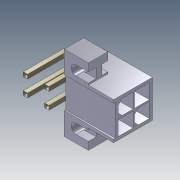
# Autodesk Inventor part: minifit-2x2rb
Saved by Autodesk Inventor 2015 SP1 (Build 190203100, 203)
## iProperties
Created: 2016-02-27
Part Number: minifit-2x2rb
Material: Generic
Document SubType Name: Modeling
Designer: Kostic
Density: 1 g/cm^3
Appearance: Default
Author: Kostic
Autodesk Inventor part; units mm, degrees
ref_plane "YZ Plane" through (0, 0, 0) normal (1, 0, 0) x (0, 1, 0)
ref_plane "XZ Plane" through (0, 0, 0) normal (0, 1, 0) x (-1, 0, 0)
ref_plane "XY Plane" through (0, 0, 0) normal (0, 0, 1) x (1, 0, 0)
sketch "Sketch1" plane through (0, 0, 0) normal (1, 0, 0) x (0, 1, 0)
  line L0 (0, 0) -> (10, 0)
  line L1 (10, 0) -> (10, -9.6)
  line L2 (10, -9.6) -> (0, -9.6)
  line L3 (0, -9.6) -> (0, 0)
  dimension "d0" = 10
  dimension "d1" = 9.6
  constraints: 8 end point, 2 parallel, 1 horizontal, 1 perpendicular
  measures "d0" distance of L1.end L2.end
  measures "d1" distance of L0.end L1.end
extrude "Extrusion1" add sketch "Sketch1" along normal blind 12.7
sketch "Sketch2" plane through (0, 0, -9.6) normal (0, -1, 0) x (1, 0, 0)
  line L0 (0, 14.55) -> (6.2, 14.55)
  line L1 (6.2, 14.55) -> (6.2, -4.95)
  line L2 (6.2, -4.95) -> (0, -4.95)
  line L3 (0, -4.95) -> (0, 14.55)
  line L4 (0, 0) -> (12.7, 0) projected
  point P0 (0, 9.6)
  dimension "d4" = 6.2
  dimension "d5" = 19.5
  dimension "d6" = 4.95
  constraints: 8 end point, 2 parallel, 1 horizontal, 1 perpendicular
  measures "d4" distance of L1.end L2.end
  measures "d5" distance of L0.end L1.end
  measures "d6" distance between parallel lines of L4 L2
extrude "Extrusion2" add sketch "Sketch2" against normal blind 5
hole "Hole1" at (3, 5, -11.3) direction (0, -1, 0) diameter 2.5 end through all
hole "Hole2" at (3, 5, 1.7) direction (0, -1, 0) diameter 2.5 end through all
sketch "Sketch3" plane through (0, 5, -9.6) normal (0, 1, 0) x (1, 0, 0)
  circle A0 centre (3, 1.7) radius 1.25 projected
  line L0 (3, 0.45) -> (6.2, 0.45)
  line L1 (6.2, 0.45) -> (6.2, 2.95)
  line L2 (6.2, 2.95) -> (3, 2.95)
  line L3 (3, 2.95) -> (3, 0.45)
  circle A1 centre (3, -11.3) radius 1.25 projected
  line L4 (3, -12.55) -> (6.2, -12.55)
  line L5 (6.2, -12.55) -> (6.2, -10.05)
  line L6 (6.2, -10.05) -> (3, -10.05)
  line L7 (3, -10.05) -> (3, -12.55)
  point P0 (0, -9.6)
  dimension "d27" = 3.2
  dimension "d28" = 2.5
  dimension "d29" = 3.2
  dimension "d30" = 2.5
  constraints: 16 end point, 4 parallel, 2 horizontal, 2 perpendicular, 2 vertical alignment, 1 point on line, 2 other
  measures "d27" distance of L2.end L1.end
  measures "d28" distance of L1.end L0.end
  measures "d29" distance of L6.end L5.end
  measures "d30" distance of L5.end L4.end
extrude "Extrusion3" cut sketch "Sketch3" against normal blind 1.5 contours A0 L3 | A0 L2 L1 L0 | A1 L7 | A1 L6 L5 L4 picked at (3.2598, 2.0258) picked at (3.5112, -11.0402)
sketch "Sketch4" plane through (12.7, 0, 0) normal (1, 0, 0) x (0, 0, -1)
  line L0 (0.8, 9.2) -> (4.6, 9.2)
  line L1 (4.6, 9.2) -> (4.6, 5.4)
  line L2 (4.6, 5.4) -> (0.8, 5.4)
  line L3 (0.8, 5.4) -> (0.8, 9.2)
  line L4 (5, 9.2) -> (8.8, 9.2)
  line L5 (8.8, 9.2) -> (8.8, 5.4)
  line L6 (8.8, 5.4) -> (5, 5.4)
  line L7 (5, 5.4) -> (5, 9.2)
  line L8 (8.8, 9.2) -> (5, 9.2)
  line L9 (5, 9.2) -> (5, 5.4)
  line L10 (5, 5.4) -> (8.8, 5.4)
  line L11 (8.8, 5.4) -> (8.8, 9.2)
  line L12 (0.8, 5) -> (4.6, 5)
  line L13 (4.6, 5) -> (4.6, 1.2)
  line L14 (4.6, 1.2) -> (0.8, 1.2)
  line L15 (0.8, 1.2) -> (0.8, 5)
  line L16 (5, 5) -> (8.8, 5)
  line L17 (8.8, 5) -> (8.8, 1.2)
  line L18 (8.8, 1.2) -> (5, 1.2)
  line L19 (5, 1.2) -> (5, 5)
  line L20 (0, 10) -> (9.6, 10) projected
  line L21 (0, 5) -> (0, 10) projected
  line L22 (9.6, 0) -> (9.6, 5) projected
  point P0 (0, 0)
  dimension "d33" = 3.8
  dimension "d34" = 3.8
  dimension "d37" = 3.8
  dimension "d39" = 3.8
  dimension "d40" = 3.8
  dimension "d43" = 0.4
  dimension "d45" = 3.8
  dimension "d46" = 3.8
  dimension "d47" = 3.8
  dimension "d52" = 0.4
  dimension "d53" = 0.4
  dimension "d118" = 0.8
  dimension "d119" = 0.8
  dimension "d120" = 0.8
  dimension "d121" = 0.8
  constraints: 40 end point, 10 parallel, 5 horizontal, 5 perpendicular, 1 point on line
  measures "d33" distance of L1.end L2.end
  measures "d34" distance of L0.end L1.end
  measures "d37" distance of L5.end L6.end
  measures "d39" distance of L10.end L9.end
  measures "d40" distance of L9.end L8.end
  measures "d43" distance between parallel lines of L1 L7
  measures "d45" distance of L13.end L14.end
  measures "d46" distance of L12.end L13.end
  measures "d47" distance of L17.end L18.end
  measures "d52" distance between parallel lines of L13 L19
  measures "d53" distance between parallel lines of L6 L16
  measures "d118" distance between parallel lines of L20 L8
  measures "d119" distance between parallel lines of L20 L0
  measures "d120" distance between parallel lines of L21 L3
  measures "d121" distance between parallel lines of L22 L17
extrude "Extrusion4" cut sketch "Sketch4" against normal blind 9
chamfer "Chamfer1" distance 1 angle 45 4 edges at (8.2, 1.2, -0.8) (8.2, 1.2, -4.6) (8.2, 5.4, -8.8) (8.2, 5.4, -5)
sketch "Sketch5" plane through (0, 10, 0) normal (0, 1, 0) x (1, 0, 0)
  line L0 (12.7, 7.8) -> (12.7, 6) projected
  line L1 (12.7, 3.3) -> (9.5, 3.3)
  line L2 (9.5, 3.3) -> (9.5, 6.3)
  line L3 (9.5, 6.3) -> (12.7, 6.3)
  line L4 (12.7, 6.3) -> (12.7, 3.3)
  line L5 (0, 9.6) -> (12.7, 9.6) projected
  point P0 (0, 0)
  point P1 (12.7, 8.8)
  point P2 (12.7, 5)
  dimension "d59" = 3.2
  dimension "d60" = 3
  dimension "d61" = 3.3
  constraints: 8 end point, 2 parallel, 1 horizontal, 1 perpendicular, 1 point on line
  measures "d59" distance of L2.end L3.end
  measures "d60" distance of L1.end L2.end
  measures "d61" distance between parallel lines of L5 L3
extrude "Extrusion5" add sketch "Sketch5" along normal blind 1.4
chamfer "Chamfer2" distance 2.8 distance2 1.4 1 edges at (12.7, 11.4, -4.8) measured on face at (12.2, 11.4, -4.8)
sketch "Sketch6" plane through (3.7, 0, 0) normal (1, 0, 0) x (0, 0, -1)
  line L0 (2.15, 7.85) -> (3.25, 7.85)
  line L1 (3.25, 7.85) -> (3.25, 6.75)
  line L2 (3.25, 6.75) -> (2.15, 6.75)
  line L3 (2.15, 6.75) -> (2.15, 7.85)
  line L4 (6.35, 7.85) -> (7.45, 7.85)
  line L5 (7.45, 7.85) -> (7.45, 6.75)
  line L6 (7.45, 6.75) -> (6.35, 6.75)
  line L7 (6.35, 6.75) -> (6.35, 7.85)
  line L8 (6.35, 7.85) -> (7.45, 7.85)
  line L9 (7.45, 7.85) -> (7.45, 6.75)
  line L10 (7.45, 6.75) -> (6.35, 6.75)
  line L11 (6.35, 6.75) -> (6.35, 7.85)
  line L12 (0.8, 5.4) -> (0.8, 9.2) projected
  line L13 (0.8, 9.2) -> (4.6, 9.2) projected
  line L14 (5, 9.2) -> (8.8, 9.2) projected
  line L15 (5, 6.4) -> (5, 9.2) projected
  line L16 (5, 6.4) -> (5, 9.2) projected
  line L17 (5, 9.2) -> (8.8, 9.2) projected
  point P0 (0, 0)
  point P1 (5, 5.4)
  point P2 (9.2, 6.4)
  dimension "d67" = 1.1
  dimension "d68" = 1.1
  dimension "d69" = 1.1
  dimension "d70" = 1.1
  dimension "d71" = 1.1
  dimension "d72" = 1.1
  dimension "d73" = 1.35
  dimension "d74" = 1.35
  dimension "d75" = 1.35
  dimension "d76" = 1.35
  dimension "d77" = 1.35
  dimension "d78" = 1.35
  constraints: 24 end point, 6 parallel, 3 horizontal, 3 perpendicular, 1 point on line, 1 other
  measures "d67" distance of L1.end L2.end
  measures "d68" distance of L0.end L1.end
  measures "d69" distance of L5.end L6.end
  measures "d70" distance of L4.end L5.end
  measures "d71" distance of L9.end L10.end
  measures "d72" distance of L8.end L9.end
  measures "d73" distance between parallel lines of L12 L3
  measures "d74" distance between parallel lines of L13 L0
  measures "d75" distance between parallel lines of L14 L4
  measures "d76" distance between parallel lines of L15 L7
  measures "d78" distance between parallel lines of L17 L8
extrude "Extrusion6" add sketch "Sketch6" along normal blind 5 and the other way blind 9.9
sketch "Sketch7" plane through (3.7, 0, 0) normal (1, 0, 0) x (0, 0, -1)
  line L0 (6.35, 3.65) -> (7.45, 3.65)
  line L1 (7.45, 3.65) -> (7.45, 2.55)
  line L2 (7.45, 2.55) -> (6.35, 2.55)
  line L3 (6.35, 2.55) -> (6.35, 3.65)
  line L4 (3.25, 3.65) -> (2.15, 3.65)
  line L5 (2.15, 3.65) -> (2.15, 2.55)
  line L6 (2.15, 2.55) -> (3.25, 2.55)
  line L7 (3.25, 2.55) -> (3.25, 3.65)
  line L8 (0.8, 2.2) -> (0.8, 5) projected
  line L9 (0.8, 5) -> (4.6, 5) projected
  line L10 (5, 1.2) -> (5, 5) projected
  point P0 (0, 0)
  point P1 (5, 2.2)
  dimension "d83" = 1.1
  dimension "d84" = 1.1
  dimension "d87" = 1.1
  dimension "d88" = 1.1
  dimension "d89" = 1.35
  dimension "d90" = 1.35
  dimension "d91" = 1.35
  constraints: 16 end point, 4 parallel, 2 horizontal, 2 perpendicular
  measures "d83" distance of L1.end L2.end
  measures "d84" distance of L0.end L1.end
  measures "d87" distance of L6.end L5.end
  measures "d88" distance of L5.end L4.end
  measures "d89" distance between parallel lines of L8 L5
  measures "d90" distance between parallel lines of L4 L9
  measures "d91" distance between parallel lines of L10 L3
extrude "Extrusion7" add sketch "Sketch7" along normal blind 5 and the other way blind 4.4
sketch "Sketch8" plane through (-0.7, 0, 0) normal (-1, 0, 0) x (0, 0, 1)
  line L0 (-6.35, 3.65) -> (-7.45, 3.65)
  line L1 (-7.45, 3.65) -> (-7.45, -3.55)
  line L2 (-7.45, -3.55) -> (-6.35, -3.55)
  line L3 (-6.35, -3.55) -> (-6.35, 3.65)
  line L4 (-2.15, 3.65) -> (-3.25, 3.65)
  line L5 (-3.25, 3.65) -> (-3.25, -3.55)
  line L6 (-3.25, -3.55) -> (-2.15, -3.55)
  line L7 (-2.15, -3.55) -> (-2.15, 3.65)
  point P0 (0, 0)
  dimension "d99" = 1.1
  dimension "d100" = 7.2
  dimension "d101" = 1.1
  dimension "d102" = 7.2
  constraints: 16 end point, 4 parallel, 2 horizontal, 2 perpendicular
  measures "d99" distance of L2.end L1.end
  measures "d100" distance of L1.end L0.end
  measures "d101" distance of L6.end L5.end
  measures "d102" distance of L5.end L4.end
extrude "Extrusion8" add sketch "Sketch8" along normal blind 1.1
sketch "Sketch9" plane through (-6.2, 0, 0) normal (-1, 0, 0) x (0, 0, 1)
  line L0 (-6.35, 7.85) -> (-7.45, 7.85)
  line L1 (-7.45, 7.85) -> (-7.45, -3.55)
  line L2 (-7.45, -3.55) -> (-6.35, -3.55)
  line L3 (-6.35, -3.55) -> (-6.35, 7.85)
  line L4 (-2.15, 7.85) -> (-3.25, 7.85)
  line L5 (-3.25, 7.85) -> (-3.25, -3.55)
  line L6 (-3.25, -3.55) -> (-2.15, -3.55)
  line L7 (-2.15, -3.55) -> (-2.15, 7.85)
  point P0 (0, 0)
  dimension "d105" = 1.1
  dimension "d106" = 11.4
  dimension "d107" = 1.1
  dimension "d108" = 11.4
  constraints: 16 end point, 4 parallel, 2 horizontal, 2 perpendicular
  measures "d105" distance of L2.end L1.end
  measures "d106" distance of L1.end L0.end
  measures "d107" distance of L6.end L5.end
  measures "d108" distance of L5.end L4.end
extrude "Extrusion9" add sketch "Sketch9" along normal blind 1.1
chamfer "Chamfer3" distance 0.3 angle 45 32 edges at (-7.3, -3.55, -6.9) (-6.75, -3.55, -7.45) (-6.75, -3.55, -6.35) (-6.2, -3.55, -6.9) (-6.75, -3.55, -3.25) (-7.3, -3.55, -2.7) (-6.75, -3.55, -2.15) (-6.2, -3.55, -2.7) (-1.8, -3.55, -2.7) (-1.25, -3.55, -2.15) (-0.7, -3.55, -2.7) (-1.25, -3.55, -3.25) (-1.25, -3.55, -6.35) (-1.8, -3.55, -6.9) (-1.25, -3.55, -7.45) (-0.7, -3.55, -6.9) (8.7, 3.1, -7.45) (8.7, 2.55, -6.9) (8.7, 3.1, -6.35) (8.7, 3.65, -6.9) (8.7, 6.75, -6.9) (8.7, 7.3, -7.45) (8.7, 7.85, -6.9) (8.7, 7.3, -6.35) (8.7, 7.3, -2.15) (8.7, 7.3, -3.25) (8.7, 6.75, -2.7) (8.7, 7.85, -2.7) (8.7, 3.1, -3.25) (8.7, 3.65, -2.7) (8.7, 2.55, -2.7) (8.7, 3.1, -2.15)
fillet "Fillet1" radius 0.8 8 edges at (-7.3, 7.85, -6.9) (-7.3, 7.85, -2.7) (-1.8, 3.65, -2.7) (-1.8, 3.65, -6.9) (-6.2, 6.75, -6.9) (-6.2, 6.75, -2.7) (-0.7, 2.55, -6.9) (-0.7, 2.55, -2.7)
sketch "Sketch10" plane through (12.7, 0, -9.6) normal (0, -1, 0) x (1, 0, 0)
  line L0 (-9.7, 12.55) -> (-6.5, 12.55)
  line L1 (-6.5, 12.55) -> (-6.5, 10.05)
  line L2 (-6.5, 10.05) -> (-9.7, 10.05)
  line L3 (-9.7, 10.05) -> (-9.7, 12.55)
  line L4 (-9.7, -0.45) -> (-6.5, -0.45)
  line L5 (-6.5, -0.45) -> (-6.5, -2.95)
  line L6 (-6.5, -2.95) -> (-9.7, -2.95)
  line L7 (-9.7, -2.95) -> (-9.7, -0.45)
  point P0 (-12.7, 9.6)
  dimension "d122" = 3.2
  dimension "d123" = 2.5
  dimension "d124" = 3.2
  dimension "d125" = 2.5
  constraints: 16 end point, 4 parallel, 2 horizontal, 2 perpendicular
  measures "d122" distance of L1.end L2.end
  measures "d123" distance of L0.end L1.end
  measures "d124" distance of L5.end L6.end
  measures "d125" distance of L4.end L5.end
extrude "Extrusion10" cut sketch "Sketch10" against normal blind 2
sketch "Sketch11" plane through (12.7, 0, -9.6) normal (0, -1, 0) x (1, 0, 0)
  line L0 (0, 9.6) -> (0, 0) projected
  line L1 (0, 8.8) -> (-12.7, 8.8)
  line L2 (-12.7, 8.8) -> (-12.7, 0.8)
  line L3 (-12.7, 0.8) -> (0, 0.8)
  line L4 (0, 0.8) -> (0, 8.8)
  line L5 (0, 0.8) -> (-9, 0.8) projected
  line L6 (-6.5, 9.6) -> (0, 9.6) projected
  line L7 (-6.5, 0) -> (0, 0) projected
  point P0 (-12.7, 9.6)
  dimension "d128" = 12.7
  dimension "d130" = 0.8
  dimension "d133" = 8
  dimension "d134" = 0.8
  constraints: 8 end point, 2 parallel, 1 horizontal, 1 perpendicular, 1 point on line
  measures "d128" distance of L3.end L2.end
  measures "d130" distance between parallel lines of L6 L1
  measures "d133" distance between parallel lines of L1 L3
  measures "d134" distance between parallel lines of L7 L3
extrude "Extrusion11" cut sketch "Sketch11" against normal blind 0.4
equation "\"d68\" = d67"
equation "\"d74\" = d73"
equation "\"d75\" = d73"
equation "\"d76\" = d73"
equation "\"d77\" = d73"
equation "\"d90\" = d89"
equation "\"d91\" = d89"
body "Solid1"
